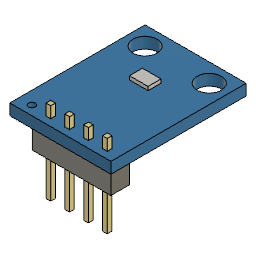
Case_Light_Sensor (Autodesk Fusion 360 archive; units mm, degrees)
design "GY-302_BH1750"
description: Open CASCADE Model
Autodesk Fusion 360 part; units mm, degrees
sketch "Sketch1" plane through (0, 0, 0) normal (0, 0, 1) x (1, 0, 0)
  line L0 (-6.825, 9.125) -> (6.825, 9.125)
  line L1 (6.825, 9.125) -> (6.825, -9.125)
  line L2 (6.825, -9.125) -> (-6.825, -9.125)
  line L3 (-6.825, -9.125) -> (-6.825, 9.125)
  circle A0 centre (-4.325, 6.625) radius 1.625
  circle A1 centre (4.325, 6.625) radius 1.625
  line L4 (-6.825, -9.125) -> (6.825, -9.125)
  line L5 (6.825, -9.125) -> (6.825, -6.625)
  line L6 (6.825, -6.625) -> (-6.825, -6.625)
  line L7 (-6.825, -6.625) -> (-6.825, -9.125)
  line L8 (-5.4, -7.555) -> (-4.76, -7.555) construction
  line L9 (-4.76, -7.555) -> (-4.76, -8.195) construction
  line L10 (-4.76, -8.195) -> (-5.4, -8.195) construction
  line L11 (-5.4, -8.195) -> (-5.4, -7.555) construction
  line L12 (-2.86, -8.195) -> (-2.86, -7.555)
  line L13 (-2.86, -7.555) -> (-2.22, -7.555)
  line L14 (-2.22, -8.195) -> (-2.86, -8.195)
  line L15 (-2.22, -7.555) -> (-2.22, -8.195)
  line L16 (-0.32, -8.195) -> (-0.32, -7.555)
  line L17 (-0.32, -7.555) -> (0.32, -7.555)
  line L18 (0.32, -8.195) -> (-0.32, -8.195)
  line L19 (0.32, -7.555) -> (0.32, -8.195)
  line L20 (2.22, -8.195) -> (2.22, -7.555)
  line L21 (2.22, -7.555) -> (2.86, -7.555)
  line L22 (2.86, -8.195) -> (2.22, -8.195)
  line L23 (2.86, -7.555) -> (2.86, -8.195)
  line L24 (4.76, -8.195) -> (4.76, -7.555)
  line L25 (4.76, -7.555) -> (5.4, -7.555)
  line L26 (5.4, -8.195) -> (4.76, -8.195)
  line L27 (5.4, -7.555) -> (5.4, -8.195)
  circle A2 centre (-5.08, -7.875) radius 0.4525
  line L28 (-3.79, -6.625) -> (-3.79, -9.125)
  line L29 (-3.79, -6.625) -> (-2.86, -7.555)
  line L30 (-1.425, 3.375) -> (1.075, 3.375)
  line L31 (1.075, 3.375) -> (1.075, 1.625)
  line L32 (1.075, 1.625) -> (-1.425, 1.625)
  line L33 (-1.425, 1.625) -> (-1.425, 3.375)
  point P0 (0, 9.125)
  point P1 (-6.825, 0)
  point P2 (-6.825, -7.875)
  point P3 (-5.4, -7.875)
  point P4 (0, -7.555)
  dimension "d1" = 3.25
  dimension "d2" = 2.5
  dimension "d3" = 2.5
  dimension "d4" = 2.5
  dimension "d5" = 18.25
  dimension "d6" = 13.65
  dimension "d7" = 2.5
  dimension "d8" = 0.64
  dimension "d11" = 2.54
  dimension "d12" = 0
  dimension "d13" = 45
  dimension "d22" = 2.5
  dimension "d23" = 5.75
  dimension "d24" = 5.75
  dimension "d25" = 1.75
  constraint horizontal L0
  constraint vertical L1
  constraint horizontal L2
  constraint vertical L3
  constraint equal A0 A1
  constraint horizontal A0.centre A1.centre
  constraint midpoint L0 P0
  constraint midpoint L3 P1
  constraint horizontal origin P1
  constraint vertical origin P0
  constraint horizontal L4
  constraint vertical L5
  constraint horizontal L6
  constraint vertical L7
  constraint coincident L1 L5.end
  constraint horizontal L8
  constraint vertical L9
  constraint horizontal L10
  constraint vertical L11
  constraint equal L8 L9
  constraint midpoint L7 P2
  constraint midpoint L11 P3
  constraint horizontal P2 P3
  constraint midpoint L17 P4
  constraint vertical origin P4
  constraint coincident L8.start A2
  constraint coincident L8.end A2
  constraint coincident L9.end A2
  constraint coincident L6 L28.start
  constraint coincident L4 L28.end
  constraint perpendicular L4 L28
  constraint horizontal L30
  constraint vertical L31
  constraint horizontal L32
  constraint vertical L33
  measures "d1" diameter of A1
  measures "d2" distance of L1 A1.centre
  measures "d3" distance of L0 A1.centre
  measures "d4" distance of L3 A0.centre
  measures "d5" distance of L0.start L2.end
  measures "d6" distance of L0.start L0.end
  measures "d7" distance of L2.end L6.end
  measures "d8" distance of L8.start L8.end
  measures "d13" angle of L6 L29
  measures "d22" distance of L30.start L30.end
  measures "d23" distance of L1 L31
  measures "d24" distance of L0 L30
  measures "d25" distance of L30.end L31.end
extrude "Extrude1" add sketch "Sketch1" against normal blind 1.5 contours L0 L1 L3 L6 | L2 L3 L4 L6 L7 L28 | L1 L2 L4 L5 L6 L28 | L30 L31 L32 L33 makes body 1
extrude "Extrude2" add sketch "Sketch1" against normal blind 11.15 from surface at 1.5 separate body contours L12 L13 L14 L15 | L16 L17 L18 L19 | L20 L21 L22 L23 | L24 L25 L26 L27 makes body 2 at (-0.32, -7.9817, -5.9333) makes body 3 at (2.22, -7.9817, -5.9333) makes body 4 at (-2.6467, -7.555, -5.9333) makes body 5 at (4.76, -7.9817, -5.9333)
extrude "Extrude3" add sketch "Sketch1" against normal blind 2.5 from surface at -1.5 separate body contours L1 L2 L4 L5 L6 L28 makes body 6
extrude "Extrude4" add sketch "Sketch1" along normal blind 0.5 separate body contours L30 L31 L32 L33 makes body 7
equation "d3 = d2"
equation "d4 = d3"
equation "d24 = d23"
